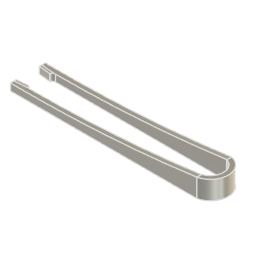
Tweezers (Autodesk Fusion 360 design; units mm, degrees)
Autodesk Fusion 360 part; units mm, degrees
sketch "Sketch1" plane through (0, 0, 0) normal (0, 0, 1) x (1, 0, 0)
  line L0 (40, 7.5) -> (-40, 7.5)
  line L1 (-40, -7.5) -> (40, -7.5)
  line L2 (40, 7.5) -> (-40, -7.5) construction
  line L3 (-40, 7.5) -> (40, -7.5) construction
  arc A0 (40, -7.5) -> (40, 7.5) centre (38.3125, 0) ccw
  line L4 (-35, -5.5) -> (39.7608, -5.5)
  arc A1 (39.7608, -5.5) -> (39.7608, 5.5) centre (38.3125, 0) ccw
  line L5 (39.7608, 5.5) -> (-35, 5.5)
  line L6 (-40, 7.5) -> (-40, 5.9374)
  line L7 (-40, -5.9374) -> (-40, -7.5)
  line L8 (-35, 5.5) -> (-40, 5.9374)
  line L9 (-35, -5.5) -> (-40, -5.9374)
  line L10 (1.75, 0) -> (22.5, 0)
  dimension "d1" = 80
  dimension "d2" = 15
  dimension "d6" = 5
  constraint horizontal L0
  constraint perpendicular L0 L6
  constraint parallel L0 L1
  constraint coincident L2 origin
  constraint coincident L3 origin
  constraint concentric A0 A1
  constraint collinear L6 L7
  constraint symmetric L8 L9 L10
  measures "d1" distance of L0.start L0.end
  measures "d2" distance of L0.end L1.start
  measures "d6" angle of L5 L8
extrude "Extrude1" add sketch "Sketch1" along normal blind 8
sketch "Sketch2" plane through (0, -7.5, 0) normal (0, -1, 0) x (1, 0, 0)
  line L0 (-40, 0) -> (40, 0)
  line L1 (40, 0) -> (40, 8)
  line L2 (40, 8) -> (-40, 8)
  line L3 (-40, 8) -> (-40, 0)
  arc A0 (-40, 3) -> (40, 8) centre (-33.4167, 540.1667) ccw
  point P0 (-40, 3)
  dimension "d9" = 3
  constraint coincident L3 P0
  constraint coincident L1.end L2.start
  constraint coincident P0 A0.start
  measures "d9" distance of L0.start P0
extrude "Extrude2" cut sketch "Sketch2" against normal through all contours L2 L3 A0
extrude "Extrude3" add 1 faces at (-37.5, -5.7187, 0.9917) along direction (-0.087156, 0.996195, 0) blind 1
extrude "Extrude4" add 1 faces at (-37.5, 5.7187, 0.9917) along direction (-0.087156, -0.996195, 0) blind 1
fillet "Fillet1" radius 1.5 1 edges at (-35, 5.5, 1.481)
fillet "Fillet2" radius 1.6 1 edges at (-35, -5.5, 1.481)
